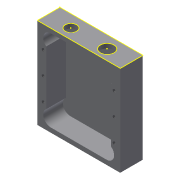
# Autodesk Inventor part: Light-tight_box
Saved by Autodesk Inventor 2015 (Build 190159000, 159)
## iProperties
Created: 2016-10-14
Part Number: Light-tight_box
Material: Generic
Document SubType Name: Modeling
Designer: HAL9000
Density: 1 g/cm^3
Appearance: Default
Author: HAL9000
Autodesk Inventor part; units mm, degrees
ref_plane "YZ Plane" through (0, 0, 0) normal (1, 0, 0) x (0, 1, 0)
ref_plane "XZ Plane" through (0, 0, 0) normal (0, 1, 0) x (-1, 0, 0)
ref_plane "XY Plane" through (0, 0, 0) normal (0, 0, 1) x (1, 0, 0)
sketch "Sketch1" plane through (0, 0, 0) normal (0, 0, 1) x (1, 0, 0)
  line L0 (0, 0) -> (69.85, 0)
  line L1 (69.85, 0) -> (69.85, 76.2)
  line L2 (69.85, 76.2) -> (0, 76.2)
  line L3 (0, 76.2) -> (0, 0)
  line L4 (0, 76.2) -> (7.62, 76.2)
  line L5 (7.62, 3.81) -> (62.23, 3.81)
  line L6 (58.42, 72.39) -> (7.62, 72.39)
  line L7 (7.62, 72.39) -> (11.43, 72.39)
  line L8 (0, 76.2) -> (69.85, 76.2)
  line L9 (34.925, 76.2) -> (50.165, 76.2)
  line L10 (50.165, 76.2) -> (50.165, 69.1676)
  line L11 (34.925, 76.2) -> (19.685, 76.2)
  line L12 (19.685, 76.2) -> (14.9225, 76.2)
  line L13 (0, 76.2) -> (0, 57.15)
  line L14 (19.685, 76.2) -> (13.9303, 76.2)
  arc A0 (11.43, 72.39) -> (7.62, 60.96) centre (11.43, 66.04) ccw
  line L15 (7.62, 3.81) -> (11.43, 3.81)
  line L16 (11.43, 3.81) -> (11.43, 10.16)
  line L17 (62.23, 3.81) -> (58.42, 3.81)
  line L18 (58.42, 3.81) -> (58.42, 10.16)
  arc A1 (7.62, 15.24) -> (11.43, 3.81) centre (11.43, 10.16) ccw
  arc A2 (58.42, 3.81) -> (62.23, 15.24) centre (58.42, 10.16) ccw
  arc A3 (62.23, 60.96) -> (58.42, 72.39) centre (58.42, 66.04) ccw
  line L19 (62.23, 15.24) -> (62.23, 60.96)
  line L20 (7.62, 60.96) -> (7.62, 15.24)
  dimension "d9" = 7.62
  dimension "d13" = 15.24
  dimension "d18" = 19.05
  dimension "d24" = 6.35
  dimension "d25" = 3.81
  dimension "d26" = 6.35
  constraints: 42 end point, 9 point on line, 8 point on circle, 4 centre point, 3 perpendicular, 2 coincident, 1 collinear, 1 horizontal, 1 midpoint, 1 tangent, 1 vertical
  measures "d9" distance of L3.start L4.end
  measures "d13" distance of L9.start L9.end
  measures "d18" distance of L3.start L13.end
  measures "d24" distance of L15.end L16.end
  measures "d25" distance of L5.end L17.end
  measures "d26" distance of L17.end L18.end
extrude "Extrusion1" add sketch "Sketch1" along normal blind 19.05
sketch "Sketch3" plane through (0, 0, 0) normal (0, 0, -1) x (-1, 0, 0)
  arc A0 (-11.43, 3.81) -> (-7.62, 15.24) centre (-11.43, 10.16) ccw projected
  line L0 (-11.43, 3.81) -> (-58.42, 3.81) projected
  arc A1 (-62.23, 15.24) -> (-58.42, 3.81) centre (-58.42, 10.16) ccw projected
  line L1 (-62.23, 15.24) -> (-62.23, 60.96) projected
  arc A2 (-58.42, 72.39) -> (-62.23, 60.96) centre (-58.42, 66.04) ccw projected
  line L2 (-58.42, 72.39) -> (-11.43, 72.39) projected
  arc A3 (-7.62, 60.96) -> (-11.43, 72.39) centre (-11.43, 66.04) ccw projected
  line L3 (-7.62, 60.96) -> (-7.62, 15.24) projected
  line L4 (0, 76.2) -> (0, 0) projected
  line L5 (-69.85, 76.2) -> (0, 76.2) projected
  line L6 (-69.85, 0) -> (-69.85, 76.2) projected
  line L7 (0, 0) -> (-69.85, 0) projected
  line L8 (0, 76.2) -> (-5.08, 76.2)
  line L9 (-69.85, 76.2) -> (0, 76.2) projected
  line L10 (-5.08, 76.2) -> (-5.08, 0)
  line L11 (-5.08, 76.2) -> (-5.08, 57.15)
  line L12 (-5.08, 0) -> (-5.08, 19.05)
  line L13 (-69.85, 0) -> (-64.77, 0)
  line L14 (0, 0) -> (-69.85, 0) projected
  line L15 (-64.77, 0) -> (-64.77, 19.05)
  line L16 (-69.85, 76.2) -> (-64.77, 76.2)
  line L17 (-64.77, 76.2) -> (-64.77, 57.15)
  line L18 (-64.77, 57.15) -> (-64.77, 38.1)
  line L19 (-5.08, 57.15) -> (-5.08, 38.1)
  dimension "d31" = 5.08
  dimension "d32" = 19.05
  dimension "d33" = 19.05
  dimension "d34" = 5.08
  dimension "d35" = 19.05
  dimension "d36" = 5.08
  dimension "d37" = 19.05
  dimension "d38" = 19.05
  dimension "d39" = 19.05
  constraints: 20 end point, 7 point on line, 6 coincident, 3 perpendicular, 1 midpoint
  measures "d31" distance of L4.start L8.end
  measures "d32" distance of L8.end L11.end
  measures "d33" distance of L10.end L12.end
  measures "d34" distance of L6.start L13.end
  measures "d35" distance of L13.end L15.end
  measures "d36" distance of L5.start L16.end
  measures "d37" distance of L16.end L17.end
  measures "d38" distance of L17.end L18.end
  measures "d39" distance of L11.end L19.end
hole "Hole1" at (64.77, 57.15, 0) at (64.77, 38.1, 0) at (64.77, 19.05, 0) at (5.08, 19.05, 0) at (5.08, 38.1, 0) at (5.08, 57.15, 0) direction (0, 0, 1) diameter 2.6416 depth 23.0124 tip angle 118 thread size "6-32 UNC" class "2B" standard "ANSI Unified Screw Threads"
sketch "Sketch7" plane through (0, 0, 0) normal (0, 0, -1) x (-1, 0, 0)
  circle A0 centre (-5.08, 38.1) radius 1.3208 projected
  circle A1 centre (-64.77, 19.05) radius 1.3208 projected
  circle A2 centre (-64.77, 57.15) radius 1.3208 projected
  circle A3 centre (-64.77, 38.1) radius 1.3208 projected
  circle A4 centre (-5.08, 19.05) radius 1.3208 projected
  circle A5 centre (-5.08, 57.15) radius 1.3208 projected
  arc A6 (-11.43, 3.81) -> (-7.62, 15.24) centre (-11.43, 10.16) ccw projected
  line L0 (-11.43, 3.81) -> (-58.42, 3.81) projected
  arc A7 (-62.23, 15.24) -> (-58.42, 3.81) centre (-58.42, 10.16) ccw projected
  line L1 (-62.23, 15.24) -> (-62.23, 60.96) projected
  arc A8 (-58.42, 72.39) -> (-62.23, 60.96) centre (-58.42, 66.04) ccw projected
  line L2 (-58.42, 72.39) -> (-11.43, 72.39) projected
  arc A9 (-7.62, 60.96) -> (-11.43, 72.39) centre (-11.43, 66.04) ccw projected
  line L3 (-7.62, 60.96) -> (-7.62, 15.24) projected
  line L4 (0, 76.2) -> (0, 0) projected
  line L5 (-69.85, 76.2) -> (0, 76.2) projected
  line L6 (-69.85, 0) -> (-69.85, 76.2) projected
  line L7 (0, 0) -> (-69.85, 0) projected
extrude "Extrusion4" add sketch "Sketch7" against normal blind 2.54 contours L0 A7 L1 A8 L2 A9 L3 A6 | L4 L7 L6 L5
sketch "Sketch8" plane through (0, 76.2, 19.05) normal (0, 1, 0) x (1, 0, 0)
  point P0 (0, 19.05)
sketch "Sketch9" plane through (0, 76.2, 19.05) normal (0, 1, 0) x (1, 0, 0)
  line L0 (0, 19.05) -> (0, 0) projected
  line L1 (69.85, 0) -> (0, 0) projected
  line L2 (69.85, 19.05) -> (69.85, 0) projected
  line L3 (69.85, 19.05) -> (0, 19.05) projected
  line L4 (0, 19.05) -> (69.85, 19.05)
  line L5 (0, 19.05) -> (69.85, 19.05) projected
  line L6 (34.925, 19.05) -> (34.925, 8.636)
  line L7 (34.925, 8.636) -> (19.685, 8.636)
  dimension "d74" = 10.414
  dimension "d75" = 15.24
  constraints: 6 end point, 1 coincident, 1 horizontal, 1 midpoint, 1 perpendicular, 1 vertical
  measures "d74" distance of L6.start L6.end
  measures "d75" distance of L6.end L7.end
hole "Hole4" at (19.685, 76.2, 10.414) direction (0, -1, 0) diameter 9.525 depth 25.4 tip angle 118
sketch "Sketch10" plane through (0, 76.2, 19.05) normal (0, 1, 0) x (1, 0, 0)
  circle A0 centre (19.685, 8.636) radius 4.7625 projected
  line L0 (0, 19.05) -> (0, 0) projected
  line L1 (69.85, 0) -> (0, 0) projected
  line L2 (69.85, 19.05) -> (69.85, 0) projected
  line L3 (69.85, 19.05) -> (0, 19.05) projected
  line L4 (69.85, 19.05) -> (0, 19.05)
  line L5 (69.85, 19.05) -> (0, 19.05) projected
  line L6 (34.925, 19.05) -> (34.925, 8.636)
  line L7 (34.925, 8.636) -> (50.165, 8.636)
  dimension "d83" = 15.24
  dimension "d91" = 10.414
  constraints: 6 end point, 1 coincident, 1 horizontal, 1 midpoint, 1 perpendicular, 1 vertical
  measures "d83" distance of L6.end L7.end
  measures "d91" distance of L6.start L6.end
hole "Hole5" at (50.165, 76.2, 10.414) direction (0, -1, 0) diameter 11.5094 depth 25.4 tip angle 118
sketch "Sketch11" plane through (0, 76.2, 19.05) normal (0, 1, 0) x (1, 0, 0)
  circle A0 centre (50.165, 8.636) radius 5.7547 projected
  circle A1 centre (19.685, 8.636) radius 4.7625 projected
  line L0 (0, 19.05) -> (0, 0) projected
  line L1 (69.85, 0) -> (0, 0) projected
  line L2 (69.85, 19.05) -> (69.85, 0) projected
  line L3 (69.85, 19.05) -> (0, 19.05) projected
body "Solid1"
